val_net_stamp (Autodesk Fusion 360 design; units mm, degrees)
Autodesk Fusion 360 part; units mm, degrees
(part 1 of 3)
sketch "Sketch1" plane through (0, 0, 0) normal (0, 1, 0) x (1, 0, 0)
  spline S0 degree 3 poles (-44.0393, 3.3032) (-46.2975, 3.0854) (-48.3436, 1.4806) (-49.1116, -0.6573) knots 0 0 0 0 1 1 1 1
  spline S1 degree 3 poles (-49.1116, -0.6573) (-49.8911, -2.841) (-49.4211, -5.145) (-47.822, -6.9218) knots 0 0 0 0 1 1 1 1
  spline S2 degree 3 poles (-47.822, -6.9218) (-46.5783, -8.3031) (-45.6555, -10.4295) (-45.1168, -13.1405) knots 0 0 0 0 1 1 1 1
  line L0 (-45.1168, -13.1405) -> (-44.985, -13.7996)
  line L1 (-44.985, -13.7996) -> (-44.9563, -26.2082)
  line L2 (-44.9563, -26.2082) -> (-44.9276, -38.6169)
  line L3 (-44.9276, -38.6169) -> (-44.7729, -39.1958)
  spline S3 degree 3 poles (-44.7729, -39.1958) (-44.492, -40.2561) (-44.2227, -40.8636) (-43.6323, -41.7405) knots 0 0 0 0 1 1 1 1
  spline S4 degree 3 poles (-43.6323, -41.7405) (-42.6924, -43.1505) (-41.0761, -44.2968) (-39.4082, -44.7438) knots 0 0 0 0 1 1 1 1
  spline S5 degree 3 poles (-39.4082, -44.7438) (-38.474, -44.996) (-38.0384, -45.019) (-34.7829, -44.996) knots 0 0 0 0 1 1 1 1
  spline S6 degree 3 poles (-34.7829, -44.996) (-31.8599, -44.9731) (-31.728, -44.9674) (-31.3498, -44.847) knots 0 0 0 0 1 1 1 1
  spline S7 degree 3 poles (-31.3498, -44.847) (-30.8626, -44.6923) (-30.3124, -44.4401) (-29.957, -44.1994) knots 0 0 0 0 1 1 1 1
  spline S8 degree 3 poles (-29.957, -44.1994) (-29.8023, -44.1019) (-27.8077, -42.1475) (-25.5208, -39.8606) knots 0 0 0 0 1 1 1 1
  spline S9 degree 3 poles (-25.5208, -39.8606) (-23.2282, -37.5795) (-21.3311, -35.7168) (-21.3025, -35.7282) knots 0 0 0 0 1 1 1 1
  spline S10 degree 3 poles (-21.3025, -35.7282) (-21.2738, -35.7397) (-19.8868, -37.1267) (-18.2247, -38.806) knots 0 0 0 0 1 1 1 1
  line L4 (-18.2247, -38.806) -> (-15.1927, -41.8552)
  line L5 (-15.1927, -41.8552) -> (-18.1674, -41.8552)
  line L6 (-18.1674, -41.8552) -> (-21.142, -41.8552)
  line L7 (-21.142, -41.8552) -> (-22.7181, -43.4313)
  line L8 (-22.7181, -43.4313) -> (-24.2943, -45.0132)
  line L9 (-24.2943, -45.0132) -> (-14.2642, -44.9903)
  spline S11 degree 3 poles (-14.2642, -44.9903) (-4.3201, -44.9731) (-4.2284, -44.9731) (-3.7183, -44.8527) knots 0 0 0 0 1 1 1 1
  spline S12 degree 3 poles (-3.7183, -44.8527) (-0.9442, -44.2108) (1.0962, -42.3997) (1.9559, -39.832) knots 0 0 0 0 1 1 1 1
  spline S13 degree 3 poles (1.9559, -39.832) (2.3514, -38.6455) (2.3284, -39.4823) (2.3284, -26.4661) knots 0 0 0 0 1 1 1 1
  spline S14 degree 3 poles (2.3284, -26.4661) (2.3284, -18.5051) (2.3456, -14.5045) (2.3915, -14.0804) knots 0 0 0 0 1 1 1 1
  spline S15 degree 3 poles (2.3915, -14.0804) (2.5577, -12.3552) (3.1079, -10.4409) (3.8587, -8.9278) knots 0 0 0 0 1 1 1 1
  spline S16 degree 3 poles (3.8587, -8.9278) (4.2714, -8.1082) (4.6669, -7.5007) (5.2171, -6.8645) knots 0 0 0 0 1 1 1 1
  spline S17 degree 3 poles (5.2171, -6.8645) (5.9966, -5.9589) (6.3978, -5.2253) (6.6672, -4.228) knots 0 0 0 0 1 1 1 1
  spline S18 degree 3 poles (6.6672, -4.228) (6.799, -3.7236) (6.8162, -3.546) (6.8219, -2.7378) knots 0 0 0 0 1 1 1 1
  spline S19 degree 3 poles (6.8219, -2.7378) (6.8219, -1.9813) (6.8047, -1.7348) (6.7015, -1.3336) knots 0 0 0 0 1 1 1 1
  spline S20 degree 3 poles (6.7015, -1.3336) (5.7043, 2.6097) (1.2624, 4.5354) (-2.2109, 2.5351) knots 0 0 0 0 1 1 1 1
  spline S21 degree 3 poles (-2.2109, 2.5351) (-3.3572, 1.8703) (-4.7843, 1.3889) (-6.2975, 1.1596) knots 0 0 0 0 1 1 1 1
  spline S22 degree 3 poles (-6.2975, 1.1596) (-7.5756, 0.9647) (-8.9167, 0.9533) (-22.145, 0.9762) knots 0 0 0 0 1 1 1 1
  spline S23 degree 3 poles (-22.145, 0.9762) (-33.9862, 0.9934) (-35.2472, 1.0048) (-35.8948, 1.0908) knots 0 0 0 0 1 1 1 1
  spline S24 degree 3 poles (-35.8948, 1.0908) (-37.6888, 1.3373) (-39.2305, 1.8302) (-40.4915, 2.5695) knots 0 0 0 0 1 1 1 1
  spline S25 degree 3 poles (-40.4915, 2.5695) (-41.4945, 3.1541) (-42.807, 3.4235) (-44.0393, 3.3032) knots 0 0 0 0 1 1 1 1
  spline S26 degree 3 poles (-10.5731, -2.2678) (-7.352, -2.841) (-5.048, -4.3484) (-3.2196, -7.0937) knots 0 0 0 0 1 1 1 1
  spline S27 degree 3 poles (-3.2196, -7.0937) (-2.4975, -8.177) (-1.6607, -9.9939) (-1.3913, -11.0657) knots 0 0 0 0 1 1 1 1
  line L10 (-1.3913, -11.0657) -> (-1.3168, -11.3694)
  line L11 (-1.3168, -11.3694) -> (-4.3717, -14.4243)
  spline S28 degree 3 poles (-4.3717, -14.4243) (-7.0483, -17.1009) (-7.4151, -17.4906) (-7.3234, -17.5422) knots 0 0 0 0 1 1 1 1
  spline S29 degree 3 poles (-7.3234, -17.5422) (-7.1342, -17.6397) (-4.492, -18.7573) (-4.4519, -18.7573) knots 0 0 0 0 1 1 1 1
  spline S30 degree 3 poles (-4.4519, -18.7573) (-4.4233, -18.7573) (-3.6037, -17.9549) (-2.6293, -16.9805) knots 0 0 0 0 1 1 1 1
  spline S31 degree 3 poles (-2.6293, -16.9805) (-1.655, -16.0005) (-0.8354, -15.2038) (-0.8124, -15.2038) knots 0 0 0 0 1 1 1 1
  spline S32 degree 3 poles (-0.8124, -15.2038) (-0.7379, -15.2038) (-0.7551, -37.5336) (-0.8296, -38.0495) knots 0 0 0 0 1 1 1 1
  spline S33 degree 3 poles (-0.8296, -38.0495) (-1.0589, -39.7173) (-2.1708, -41.07) (-3.7871, -41.6488) knots 0 0 0 0 1 1 1 1
  line L12 (-3.7871, -41.6488) -> (-4.2914, -41.8265)
  line L13 (-4.2914, -41.8265) -> (-7.5584, -41.8437)
  line L14 (-7.5584, -41.8437) -> (-10.8196, -41.8609)
  line L15 (-10.8196, -41.8609) -> (-14.9921, -37.6884)
  line L16 (-14.9921, -37.6884) -> (-19.1646, -33.5159)
  line L17 (-19.1646, -33.5159) -> (-15.1411, -29.4924)
  spline S34 degree 3 poles (-15.1411, -29.4924) (-12.923, -27.2743) (-11.0947, -25.4689) (-11.0718, -25.4746) knots 0 0 0 0 1 1 1 1
  spline S35 degree 3 poles (-11.0718, -25.4746) (-11.0489, -25.4861) (-9.4842, -27.0336) (-7.5928, -28.9192) knots 0 0 0 0 1 1 1 1
  line L18 (-7.5928, -28.9192) -> (-4.1481, -32.3466)
  line L19 (-4.1481, -32.3466) -> (-4.1481, -30.1801)
  line L20 (-4.1481, -30.1801) -> (-4.1481, -28.0136)
  line L21 (-4.1481, -28.0136) -> (-11.6564, -20.5054)
  line L22 (-11.6564, -20.5054) -> (-19.1646, -12.9972)
  line L23 (-19.1646, -12.9972) -> (-15.4334, -9.266)
  line L24 (-15.4334, -9.266) -> (-11.7022, -5.5348)
  line L25 (-11.7022, -5.5348) -> (-12.6651, -5.5004)
  spline S36 degree 3 poles (-12.6651, -5.5004) (-13.1924, -5.4775) (-14.1496, -5.4603) (-14.7858, -5.4603) knots 0 0 0 0 1 1 1 1
  line L26 (-14.7858, -5.4603) -> (-15.955, -5.4603)
  line L27 (-15.955, -5.4603) -> (-18.6029, -8.1254)
  spline S37 degree 3 poles (-18.6029, -8.1254) (-20.053, -9.5927) (-21.2738, -10.7905) (-21.3082, -10.7905) knots 0 0 0 0 1 1 1 1
  spline S38 degree 3 poles (-21.3082, -10.7905) (-21.3426, -10.7905) (-22.3743, -9.7933) (-23.6008, -8.5667) knots 0 0 0 0 1 1 1 1
  spline S39 degree 3 poles (-23.6008, -8.5667) (-24.8216, -7.3459) (-25.8361, -6.3716) (-25.8475, -6.406) knots 0 0 0 0 1 1 1 1
  spline S40 degree 3 poles (-25.8475, -6.406) (-25.8647, -6.4346) (-26.157, -7.1224) (-26.5009, -7.9248) knots 0 0 0 0 1 1 1 1
  line L28 (-26.5009, -7.9248) -> (-27.1257, -9.3863)
  line L29 (-27.1257, -9.3863) -> (-20.1791, -16.3329)
  line L30 (-20.1791, -16.3329) -> (-13.2325, -23.2852)
  line L31 (-13.2325, -23.2852) -> (-17.2732, -27.3259)
  line L32 (-17.2732, -27.3259) -> (-21.3139, -31.3666)
  line L33 (-21.3139, -31.3666) -> (-23.5607, -29.1198)
  line L34 (-23.5607, -29.1198) -> (-25.8074, -26.8731)
  line L35 (-25.8074, -26.8731) -> (-25.9278, -27.1597)
  spline S41 degree 3 poles (-25.9278, -27.1597) (-25.9966, -27.3144) (-26.2831, -27.9907) (-26.5697, -28.6613) knots 0 0 0 0 1 1 1 1
  line L36 (-26.5697, -28.6613) -> (-27.0913, -29.8878)
  line L37 (-27.0913, -29.8878) -> (-25.3088, -31.6703)
  spline S42 degree 3 poles (-25.3088, -31.6703) (-24.323, -32.6561) (-23.5206, -33.4872) (-23.5206, -33.5159) knots 0 0 0 0 1 1 1 1
  spline S43 degree 3 poles (-23.5206, -33.5159) (-23.5206, -33.5503) (-25.3088, -35.3557) (-27.4867, -37.5336) knots 0 0 0 0 1 1 1 1
  spline S44 degree 3 poles (-27.4867, -37.5336) (-31.195, -41.2304) (-31.4816, -41.4998) (-31.8312, -41.6603) knots 0 0 0 0 1 1 1 1
  line L38 (-31.8312, -41.6603) -> (-32.2037, -41.8265)
  line L39 (-32.2037, -41.8265) -> (-35.0924, -41.8437)
  spline S45 degree 3 poles (-35.0924, -41.8437) (-38.3708, -41.8609) (-38.4568, -41.8494) (-39.3681, -41.4024) knots 0 0 0 0 1 1 1 1
  spline S46 degree 3 poles (-39.3681, -41.4024) (-40.4399, -40.8694) (-41.185, -40.0039) (-41.6148, -38.7888) knots 0 0 0 0 1 1 1 1
  line L40 (-41.6148, -38.7888) -> (-41.7753, -38.3303)
  line L41 (-41.7753, -38.3303) -> (-41.7925, -26.7928)
  spline S47 degree 3 poles (-41.7925, -26.7928) (-41.7982, -20.4538) (-41.7868, -15.2611) (-41.7639, -15.2611) knots 0 0 0 0 1 1 1 1
  spline S48 degree 3 poles (-41.7639, -15.2611) (-41.6951, -15.2611) (-33.7799, -23.1877) (-33.7799, -23.2565) knots 0 0 0 0 1 1 1 1
  spline S49 degree 3 poles (-33.7799, -23.2565) (-33.7799, -23.2909) (-34.8345, -24.3742) (-36.1298, -25.6637) knots 0 0 0 0 1 1 1 1
  line L42 (-36.1298, -25.6637) -> (-38.4797, -28.0136)
  line L43 (-38.4797, -28.0136) -> (-38.4797, -30.1801)
  line L44 (-38.4797, -30.1801) -> (-38.4797, -32.3466)
  line L45 (-38.4797, -32.3466) -> (-32.0261, -25.8701)
  spline S50 degree 3 poles (-32.0261, -25.8701) (-28.4783, -22.3108) (-25.5724, -19.3763) (-25.5724, -19.3534) knots 0 0 0 0 1 1 1 1
  spline S51 degree 3 poles (-25.5724, -19.3534) (-25.5724, -19.3133) (-27.5956, -18.4249) (-28.3235, -18.144) knots 0 0 0 0 1 1 1 1
  line L46 (-28.3235, -18.144) -> (-28.5757, -18.0523)
  line L47 (-28.5757, -18.0523) -> (-30.0888, -19.5654)
  line L48 (-30.0888, -19.5654) -> (-31.6019, -21.0786)
  line L49 (-31.6019, -21.0786) -> (-36.4508, -16.2297)
  line L50 (-36.4508, -16.2297) -> (-41.2939, -11.3866)
  line L51 (-41.2939, -11.3866) -> (-41.1105, -10.8192)
  spline S52 degree 3 poles (-41.1105, -10.8192) (-40.5087, -8.9278) (-39.6203, -7.2542) (-38.5141, -5.9303) knots 0 0 0 0 1 1 1 1
  spline S53 degree 3 poles (-38.5141, -5.9303) (-37.9868, -5.2941) (-37.1615, -4.526) (-36.5024, -4.0503) knots 0 0 0 0 1 1 1 1
  spline S54 degree 3 poles (-36.5024, -4.0503) (-35.8891, -3.6147) (-34.588, -2.9499) (-33.8659, -2.7149) knots 0 0 0 0 1 1 1 1
  spline S55 degree 3 poles (-33.8659, -2.7149) (-33.1896, -2.4914) (-32.0031, -2.2506) (-31.2867, -2.1933) knots 0 0 0 0 1 1 1 1
  spline S56 degree 3 poles (-31.2867, -2.1933) (-30.9715, -2.1704) (-26.3003, -2.1532) (-20.9127, -2.1647) knots 0 0 0 0 1 1 1 1
  spline S57 degree 3 poles (-20.9127, -2.1647) (-12.0748, -2.1704) (-11.0603, -2.1819) (-10.5731, -2.2678) knots 0 0 0 0 1 1 1 1
extrude "Extrude1" add sketch "Sketch1" against normal blind 12 makes body 1
sketch "Sketch2" plane through (0, 0, 0) normal (0, 1, 0) x (1, 0, 0)
  spline S0 degree 3 poles (34.0518, 3.2009) (31.7591, 2.9797) (29.6817, 1.3504) (28.902, -0.8201) knots 0 0 0 0 1 1 1 1
  spline S1 degree 3 poles (28.902, -0.8201) (28.1106, -3.0372) (28.5877, -5.3764) (30.2112, -7.1803) knots 0 0 0 0 1 1 1 1
  spline S2 degree 3 poles (30.2112, -7.1803) (31.474, -8.5827) (32.4108, -10.7416) (32.9578, -13.494) knots 0 0 0 0 1 1 1 1
  line L0 (32.9578, -13.494) -> (33.0917, -14.1632)
  line L1 (33.0917, -14.1632) -> (33.1208, -26.7614)
  line L2 (33.1208, -26.7614) -> (33.1499, -39.3597)
  line L3 (33.1499, -39.3597) -> (33.307, -39.9474)
  spline S3 degree 3 poles (33.307, -39.9474) (33.5921, -41.0239) (33.8656, -41.6407) (34.465, -42.531) knots 0 0 0 0 1 1 1 1
  spline S4 degree 3 poles (34.465, -42.531) (35.4193, -43.9625) (37.0603, -45.1263) (38.7536, -45.5802) knots 0 0 0 0 1 1 1 1
  spline S5 degree 3 poles (38.7536, -45.5802) (39.7021, -45.8363) (40.1444, -45.8595) (43.4496, -45.8363) knots 0 0 0 0 1 1 1 1
  spline S6 degree 3 poles (43.4496, -45.8363) (46.4173, -45.813) (46.5511, -45.8072) (46.9352, -45.685) knots 0 0 0 0 1 1 1 1
  spline S7 degree 3 poles (46.9352, -45.685) (47.4298, -45.5278) (47.9884, -45.2718) (48.3492, -45.0274) knots 0 0 0 0 1 1 1 1
  spline S8 degree 3 poles (48.3492, -45.0274) (48.5063, -44.9285) (50.5313, -42.9442) (52.8531, -40.6224) knots 0 0 0 0 1 1 1 1
  spline S9 degree 3 poles (52.8531, -40.6224) (55.1808, -38.3064) (57.1069, -36.4152) (57.136, -36.4269) knots 0 0 0 0 1 1 1 1
  spline S10 degree 3 poles (57.136, -36.4269) (57.1651, -36.4385) (58.5733, -37.8467) (60.2608, -39.5517) knots 0 0 0 0 1 1 1 1
  line L4 (60.2608, -39.5517) -> (63.3391, -42.6474)
  line L5 (63.3391, -42.6474) -> (60.319, -42.6474)
  line L6 (60.319, -42.6474) -> (57.2989, -42.6474)
  line L7 (57.2989, -42.6474) -> (55.6987, -44.2477)
  line L8 (55.6987, -44.2477) -> (54.0984, -45.8537)
  line L9 (54.0984, -45.8537) -> (64.2818, -45.8304)
  spline S11 degree 3 poles (64.2818, -45.8304) (74.3778, -45.813) (74.4709, -45.813) (74.9888, -45.6908) knots 0 0 0 0 1 1 1 1
  spline S12 degree 3 poles (74.9888, -45.6908) (77.8052, -45.039) (79.8768, -43.2002) (80.7497, -40.5933) knots 0 0 0 0 1 1 1 1
  spline S13 degree 3 poles (80.7497, -40.5933) (81.1512, -39.3887) (81.1279, -40.2383) (81.1279, -27.0233) knots 0 0 0 0 1 1 1 1
  spline S14 degree 3 poles (81.1279, -27.0233) (81.1279, -18.9406) (81.1454, -14.8789) (81.1919, -14.4483) knots 0 0 0 0 1 1 1 1
  spline S15 degree 3 poles (81.1919, -14.4483) (81.3607, -12.6968) (81.9193, -10.7532) (82.6816, -9.217) knots 0 0 0 0 1 1 1 1
  spline S16 degree 3 poles (82.6816, -9.217) (83.1006, -8.3849) (83.5021, -7.768) (84.0607, -7.1221) knots 0 0 0 0 1 1 1 1
  spline S17 degree 3 poles (84.0607, -7.1221) (84.8521, -6.2027) (85.2594, -5.4579) (85.5329, -4.4454) knots 0 0 0 0 1 1 1 1
  spline S18 degree 3 poles (85.5329, -4.4454) (85.6668, -3.9333) (85.6842, -3.7529) (85.69, -2.9324) knots 0 0 0 0 1 1 1 1
  spline S19 degree 3 poles (85.69, -2.9324) (85.69, -2.1643) (85.6726, -1.9141) (85.5678, -1.5068) knots 0 0 0 0 1 1 1 1
  spline S20 degree 3 poles (85.5678, -1.5068) (84.5553, 2.4967) (80.0456, 4.4519) (76.5192, 2.4211) knots 0 0 0 0 1 1 1 1
  spline S21 degree 3 poles (76.5192, 2.4211) (75.3554, 1.7461) (73.9065, 1.2573) (72.3702, 1.0245) knots 0 0 0 0 1 1 1 1
  spline S22 degree 3 poles (72.3702, 1.0245) (71.0726, 0.8267) (69.7109, 0.815) (56.2806, 0.8383) knots 0 0 0 0 1 1 1 1
  spline S23 degree 3 poles (56.2806, 0.8383) (44.2584, 0.8558) (42.9782, 0.8674) (42.3207, 0.9547) knots 0 0 0 0 1 1 1 1
  spline S24 degree 3 poles (42.3207, 0.9547) (40.4993, 1.2049) (38.934, 1.7054) (37.6538, 2.456) knots 0 0 0 0 1 1 1 1
  spline S25 degree 3 poles (37.6538, 2.456) (36.6355, 3.0496) (35.3029, 3.3231) (34.0518, 3.2009) knots 0 0 0 0 1 1 1 1
  spline S26 degree 3 poles (68.0292, -2.4553) (71.2995, -3.0372) (73.6388, -4.5676) (75.4951, -7.3549) knots 0 0 0 0 1 1 1 1
  spline S27 degree 3 poles (75.4951, -7.3549) (76.2283, -8.4547) (77.0778, -10.2993) (77.3513, -11.3875) knots 0 0 0 0 1 1 1 1
  line L10 (77.3513, -11.3875) -> (77.427, -11.6959)
  line L11 (77.427, -11.6959) -> (74.3254, -14.7975)
  spline S28 degree 3 poles (74.3254, -14.7975) (71.6079, -17.515) (71.2355, -17.9106) (71.3286, -17.963) knots 0 0 0 0 1 1 1 1
  spline S29 degree 3 poles (71.3286, -17.963) (71.5206, -18.0619) (74.2032, -19.1967) (74.244, -19.1967) knots 0 0 0 0 1 1 1 1
  spline S30 degree 3 poles (74.244, -19.1967) (74.2731, -19.1967) (75.1052, -18.382) (76.0944, -17.3928) knots 0 0 0 0 1 1 1 1
  spline S31 degree 3 poles (76.0944, -17.3928) (77.0837, -16.3977) (77.9158, -15.5888) (77.9391, -15.5888) knots 0 0 0 0 1 1 1 1
  spline S32 degree 3 poles (77.9391, -15.5888) (78.0147, -15.5888) (77.9972, -38.2599) (77.9216, -38.7836) knots 0 0 0 0 1 1 1 1
  spline S33 degree 3 poles (77.9216, -38.7836) (77.6888, -40.4769) (76.5599, -41.8502) (74.919, -42.4379) knots 0 0 0 0 1 1 1 1
  line L12 (74.919, -42.4379) -> (74.4069, -42.6183)
  line L13 (74.4069, -42.6183) -> (71.09, -42.6358)
  line L14 (71.09, -42.6358) -> (67.779, -42.6532)
  line L15 (67.779, -42.6532) -> (63.5427, -38.417)
  line L16 (63.5427, -38.417) -> (59.3065, -34.1807)
  line L17 (59.3065, -34.1807) -> (63.3914, -30.0957)
  spline S34 degree 3 poles (63.3914, -30.0957) (65.6434, -27.8438) (67.4997, -26.0108) (67.523, -26.0166) knots 0 0 0 0 1 1 1 1
  spline S35 degree 3 poles (67.523, -26.0166) (67.5462, -26.0282) (69.1348, -27.5994) (71.0551, -29.5138) knots 0 0 0 0 1 1 1 1
  line L18 (71.0551, -29.5138) -> (74.5524, -32.9936)
  line L19 (74.5524, -32.9936) -> (74.5524, -30.794)
  line L20 (74.5524, -30.794) -> (74.5524, -28.5944)
  line L21 (74.5524, -28.5944) -> (66.9294, -20.9715)
  line L22 (66.9294, -20.9715) -> (59.3065, -13.3485)
  line L23 (59.3065, -13.3485) -> (63.0947, -9.5603)
  line L24 (63.0947, -9.5603) -> (66.8829, -5.7721)
  line L25 (66.8829, -5.7721) -> (65.9053, -5.7372)
  spline S36 degree 3 poles (65.9053, -5.7372) (65.3699, -5.7139) (64.3981, -5.6965) (63.7522, -5.6965) knots 0 0 0 0 1 1 1 1
  line L26 (63.7522, -5.6965) -> (62.5651, -5.6965)
  line L27 (62.5651, -5.6965) -> (59.8767, -8.4023)
  spline S37 degree 3 poles (59.8767, -8.4023) (58.4045, -9.892) (57.1651, -11.1082) (57.1301, -11.1082) knots 0 0 0 0 1 1 1 1
  spline S38 degree 3 poles (57.1301, -11.1082) (57.0952, -11.1082) (56.0478, -10.0957) (54.8025, -8.8504) knots 0 0 0 0 1 1 1 1
  spline S39 degree 3 poles (54.8025, -8.8504) (53.5631, -7.6109) (52.5331, -6.6217) (52.5215, -6.6566) knots 0 0 0 0 1 1 1 1
  spline S40 degree 3 poles (52.5215, -6.6566) (52.504, -6.6857) (52.2072, -7.384) (51.8581, -8.1987) knots 0 0 0 0 1 1 1 1
  line L28 (51.8581, -8.1987) -> (51.2238, -9.6825)
  line L29 (51.2238, -9.6825) -> (58.2765, -16.7352)
  line L30 (58.2765, -16.7352) -> (65.3292, -23.7937)
  line L31 (65.3292, -23.7937) -> (61.2268, -27.8961)
  line L32 (61.2268, -27.8961) -> (57.1243, -31.9986)
  line L33 (57.1243, -31.9986) -> (54.8433, -29.7175)
  line L34 (54.8433, -29.7175) -> (52.5622, -27.4364)
  line L35 (52.5622, -27.4364) -> (52.44, -27.7274)
  spline S41 degree 3 poles (52.44, -27.7274) (52.3702, -27.8845) (52.0792, -28.5711) (51.7883, -29.252) knots 0 0 0 0 1 1 1 1
  line L36 (51.7883, -29.252) -> (51.2587, -30.4972)
  line L37 (51.2587, -30.4972) -> (53.0685, -32.307)
  spline S42 degree 3 poles (53.0685, -32.307) (54.0693, -33.3078) (54.884, -34.1516) (54.884, -34.1807) knots 0 0 0 0 1 1 1 1
  spline S43 degree 3 poles (54.884, -34.1807) (54.884, -34.2156) (53.0685, -36.0486) (50.8572, -38.2599) knots 0 0 0 0 1 1 1 1
  spline S44 degree 3 poles (50.8572, -38.2599) (47.0923, -42.0131) (46.8013, -42.2866) (46.4464, -42.4496) knots 0 0 0 0 1 1 1 1
  line L38 (46.4464, -42.4496) -> (46.0681, -42.6183)
  line L39 (46.0681, -42.6183) -> (43.1353, -42.6358)
  spline S45 degree 3 poles (43.1353, -42.6358) (39.8068, -42.6532) (39.7196, -42.6416) (38.7943, -42.1877) knots 0 0 0 0 1 1 1 1
  spline S46 degree 3 poles (38.7943, -42.1877) (37.7062, -41.6465) (36.9497, -40.7679) (36.5133, -39.5342) knots 0 0 0 0 1 1 1 1
  line L40 (36.5133, -39.5342) -> (36.3503, -39.0687)
  line L41 (36.3503, -39.0687) -> (36.3329, -27.355)
  spline S47 degree 3 poles (36.3329, -27.355) (36.3271, -20.9191) (36.3387, -15.647) (36.362, -15.647) knots 0 0 0 0 1 1 1 1
  spline S48 degree 3 poles (36.362, -15.647) (36.4318, -15.647) (44.4679, -23.6948) (44.4679, -23.7646) knots 0 0 0 0 1 1 1 1
  spline S49 degree 3 poles (44.4679, -23.7646) (44.4679, -23.7995) (43.3972, -24.8993) (42.0821, -26.2086) knots 0 0 0 0 1 1 1 1
  line L42 (42.0821, -26.2086) -> (39.6963, -28.5944)
  line L43 (39.6963, -28.5944) -> (39.6963, -30.794)
  line L44 (39.6963, -30.794) -> (39.6963, -32.9936)
  line L45 (39.6963, -32.9936) -> (46.2485, -26.4181)
  spline S50 degree 3 poles (46.2485, -26.4181) (49.8505, -22.8045) (52.8008, -19.8251) (52.8008, -19.8018) knots 0 0 0 0 1 1 1 1
  spline S51 degree 3 poles (52.8008, -19.8018) (52.8008, -19.7611) (50.7467, -18.8592) (50.0076, -18.574) knots 0 0 0 0 1 1 1 1
  line L46 (50.0076, -18.574) -> (49.7516, -18.4809)
  line L47 (49.7516, -18.4809) -> (48.2154, -20.0171)
  line L48 (48.2154, -20.0171) -> (46.6791, -21.5534)
  line L49 (46.6791, -21.5534) -> (41.7562, -16.6305)
  line L50 (41.7562, -16.6305) -> (36.8391, -11.7134)
  line L51 (36.8391, -11.7134) -> (37.0253, -11.1373)
  spline S52 degree 3 poles (37.0253, -11.1373) (37.6363, -9.217) (38.5383, -7.5178) (39.6614, -6.1736) knots 0 0 0 0 1 1 1 1
  spline S53 degree 3 poles (39.6614, -6.1736) (40.1967, -5.5277) (41.0347, -4.748) (41.7039, -4.265) knots 0 0 0 0 1 1 1 1
  spline S54 degree 3 poles (41.7039, -4.265) (42.3265, -3.8227) (43.6474, -3.1477) (44.3806, -2.9091) knots 0 0 0 0 1 1 1 1
  spline S55 degree 3 poles (44.3806, -2.9091) (45.0673, -2.6822) (46.2718, -2.4378) (46.9992, -2.3796) knots 0 0 0 0 1 1 1 1
  spline S56 degree 3 poles (46.9992, -2.3796) (47.3192, -2.3563) (52.0618, -2.3389) (57.5317, -2.3505) knots 0 0 0 0 1 1 1 1
  spline S57 degree 3 poles (57.5317, -2.3505) (66.5046, -2.3563) (67.5346, -2.368) (68.0292, -2.4553) knots 0 0 0 0 1 1 1 1
  line L52 (28.5927, -14.6139) -> (28.6208, -26.7718)
  line L53 (28.6208, -26.7718) -> (28.6512, -39.9559)
  line L54 (28.6512, -39.9559) -> (28.9596, -41.1095)
  spline S58 degree 3 poles (28.9596, -41.1095) (29.1624, -41.8737) (29.4207, -42.6577) (29.7867, -43.4188) (30.0662, -43.9999) (30.3895, -44.5347) (30.7268, -45.0362) knots 0.002463 0.002463 0.002463 0.002463 0.566846 0.566846 0.566846 0.997755 0.997755 0.997755 0.997755
  spline S59 degree 3 poles (30.7268, -45.0362) (31.8623, -46.7358) (33.3627, -48.0126) (35.086, -48.9323) (35.8654, -49.3483) (36.6957, -49.6868) (37.5808, -49.9247) knots 0.001217 0.001217 0.001217 0.001217 0.688337 0.688337 0.688337 0.9991 0.9991 0.9991 0.9991
  spline S60 degree 3 poles (37.5809, -49.9247) (38.1393, -50.0755) (38.9538, -50.2376) (39.748, -50.2925) (40.6559, -50.3552) (41.5987, -50.3487) (43.2784, -50.3375) knots 0 0 0 0 0.456967 0.456967 0.456967 0.979343 0.979343 0.979343 0.979343
  line L55 (43.2784, -50.3375) -> (43.2375, -50.3785)
  line L56 (43.2375, -50.3785) -> (64.2895, -50.3304)
  spline S61 degree 3 poles (64.2895, -50.3304) (69.3375, -50.3217) (71.8718, -50.3178) (73.2853, -50.2995) (73.992, -50.2904) (74.4136, -50.2812) (74.8445, -50.2498) (75.1344, -50.2286) (75.4759, -50.185) (75.7431, -50.1318) (75.8658, -50.1074) (75.9593, -50.0853) (76.0131, -50.0726) knots 0 0 0 0 0.5 0.5 0.5 0.75 0.75 0.75 0.918213 0.918213 0.918213 0.99543 0.99543 0.99543 0.99543
  spline S62 degree 3 poles (76.0131, -50.0726) (78.7497, -49.4373) (81.2312, -47.9496) (82.9657, -45.7927) (83.8624, -44.6776) (84.5567, -43.3962) (85.0168, -42.022) (85.0171, -42.0211) (85.0175, -42.0201) (85.0178, -42.0192) knots 0.000788 0.000788 0.000788 0.000788 0.659473 0.659473 0.659473 1 1 1 1.000365 1.000365 1.000365 1.000365
  spline S63 degree 3 poles (85.0178, -42.0192) (85.0181, -42.0182) (85.0184, -42.0173) (85.0187, -42.0163) (85.0516, -41.9176) (85.1158, -41.7567) (85.2177, -41.4143) (85.3321, -41.0296) (85.439, -40.5049) (85.4918, -40.0367) (85.5914, -39.1525) (85.6029, -38.2865) (85.6162, -36.5721) (85.6311, -34.6649) (85.6279, -31.7431) (85.6279, -27.0233) knots -0.000791 -0.000791 -0.000791 -0.000791 0 0 0 0.151411 0.151411 0.151411 0.321524 0.321524 0.321524 0.642699 0.642699 0.642699 1 1 1 1
  spline S64 degree 3 poles (85.6279, -27.0233) (85.6279, -23.1991) (85.6318, -20.2771) (85.6408, -18.2245) (85.6454, -17.1759) (85.6514, -16.3534) (85.6586, -15.7622) (85.664, -15.321) (85.6707, -15.0001) (85.6757, -14.8547) (85.6761, -14.8429) (85.6765, -14.8324) (85.6768, -14.8233) knots 0 0 0 0 0.473518 0.473518 0.473518 0.715422 0.715422 0.715422 0.895914 0.895914 0.895914 0.91057 0.91057 0.91057 0.91057
  spline S65 degree 3 poles (85.6768, -14.8233) (85.78, -13.825) (86.1372, -12.4963) (86.5583, -11.5465) (86.6077, -11.435) (86.6576, -11.3286) (86.707, -11.2286) knots 0.016663 0.016663 0.016663 0.016663 0.893157 0.893157 0.893157 0.99609 0.99609 0.99609 0.99609
  spline S66 degree 3 poles (86.707, -11.2286) (87.0043, -10.6397) (87.1373, -10.444) (87.4643, -10.0658) (87.4655, -10.0645) (87.4666, -10.0631) (87.4678, -10.0618) knots 0.006764 0.006764 0.006764 0.006764 1 1 1 1.002067 1.002067 1.002067 1.002067
  spline S67 degree 3 poles (87.4678, -10.0618) (87.4689, -10.0605) (87.4701, -10.0591) (87.4712, -10.0578) (88.1686, -9.2476) (88.815, -8.3206) (89.28, -7.2967) (89.5333, -6.7388) (89.7284, -6.1697) (89.8772, -5.6188) (89.8788, -5.6129) (89.8804, -5.607) (89.882, -5.6011) knots -0.001455 -0.001455 -0.001455 -0.001455 0 0 0 0.647342 0.647342 0.647342 1 1 1 1.005845 1.005845 1.005845 1.005845
  spline S68 degree 3 poles (89.882, -5.6011) (89.8836, -5.5951) (89.8851, -5.5892) (89.8867, -5.5833) (89.9571, -5.3137) (90.0431, -4.9596) (90.1002, -4.5568) (90.1621, -4.1205) (90.1782, -3.7263) (90.185, -3.3701) (90.1876, -3.2384) (90.1889, -3.1062) (90.1899, -2.9643) (90.19, -2.959) (90.19, -2.9537) (90.19, -2.9484) knots -0.011583 -0.011583 -0.011583 -0.011583 0 0 0 0.402629 0.402629 0.402629 0.838702 0.838702 0.838702 1 1 1 1.006483 1.006483 1.006483 1.006483
  spline S69 degree 3 poles (90.19, -2.9484) (90.19, -2.9431) (90.19, -2.9377) (90.19, -2.9324) (90.19, -2.4687) (90.1909, -2.0734) (90.1389, -1.562) (90.0975, -1.1547) (90.0104, -0.7153) (89.9283, -0.3949) knots -0.006925 -0.006925 -0.006925 -0.006925 0 0 0 0.554445 0.554445 0.554445 0.995951 0.995951 0.995951 0.995951
  spline S70 degree 3 poles (89.9283, -0.3949) (89.2588, 2.2434) (87.6414, 4.4379) (85.5824, 5.8498) (83.3601, 7.3736) (80.5963, 8.0488) (77.8293, 7.5933) (76.6106, 7.3927) (75.3981, 6.9683) (74.2734, 6.3206) (74.2714, 6.3195) (74.2694, 6.3184) (74.2674, 6.3172) knots 0.000423 0.000423 0.000423 0.000423 0.3917 0.3917 0.3917 0.814004 0.814004 0.814004 1 1 1 1.000565 1.000565 1.000565 1.000565
  spline S71 degree 3 poles (74.2674, 6.3172) (74.2655, 6.316) (74.2635, 6.3149) (74.2615, 6.3137) (73.6843, 5.979) (72.7241, 5.6295) (71.6961, 5.4737) (71.6954, 5.4736) (71.6947, 5.4735) (71.694, 5.4734) knots -0.00171 -0.00171 -0.00171 -0.00171 0 0 0 1 1 1 1.000449 1.000449 1.000449 1.000449
  spline S72 degree 3 poles (71.694, 5.4734) (71.6933, 5.4733) (71.6927, 5.4732) (71.692, 5.4731) (71.4636, 5.4383) (71.3375, 5.4212) (70.8719, 5.3978) (69.9429, 5.351) (67.867, 5.3283) (63.1123, 5.3297) (61.2764, 5.3303) (59.0354, 5.3336) (56.2884, 5.3383) (56.2882, 5.3383) (56.2879, 5.3383) (56.2877, 5.3383) knots -0.000531 -0.000531 -0.000531 -0.000531 0 0 0 0.265563 0.265563 0.265563 0.795413 0.795413 0.795413 1 1 1 1.000016 1.000016 1.000016 1.000016
  spline S73 degree 3 poles (56.2877, 5.3383) (56.2875, 5.3383) (56.2873, 5.3383) (56.2871, 5.3383) (49.133, 5.3487) (45.769, 5.3576) (44.1594, 5.38) (43.3075, 5.3919) (42.958, 5.4118) (42.9119, 5.4159) (42.911, 5.416) (42.9103, 5.416) (42.9096, 5.4161) knots -0.000018 -0.000018 -0.000018 -0.000018 0 0 0 0.595196 0.595196 0.595196 0.910216 0.910216 0.910216 0.916088 0.916088 0.916088 0.916088
  spline S74 degree 3 poles (42.9096, 5.4161) (41.5575, 5.6043) (40.5785, 5.9576) (39.93, 6.3379) (39.9283, 6.3389) (39.9266, 6.3399) (39.9249, 6.3409) knots 0.005759 0.005759 0.005759 0.005759 1 1 1 1.001321 1.001321 1.001321 1.001321
  spline S75 degree 3 poles (39.9249, 6.3409) (39.9232, 6.3419) (39.9215, 6.3428) (39.9198, 6.3438) (38.3615, 7.2521) (36.7048, 7.6682) (34.9959, 7.7237) (34.5397, 7.7385) (34.079, 7.7249) (33.6144, 7.6795) knots -0.001663 -0.001663 -0.001663 -0.001663 0 0 0 0.789303 0.789303 0.789303 1 1 1 1
  spline S76 degree 3 poles (33.6144, 7.6795) (31.0087, 7.4269) (28.7159, 6.2217) (27.0024, 4.4425) (25.9971, 3.3987) (25.1834, 2.1388) (24.6669, 0.7013) (24.6659, 0.6984) (24.6649, 0.6956) (24.6639, 0.6927) knots 0.000439 0.000439 0.000439 0.000439 0.630416 0.630416 0.630416 1 1 1 1.001322 1.001322 1.001322 1.001322
  spline S77 degree 3 poles (24.6639, 0.6927) (23.792, -1.7499) (23.8315, -4.463) (24.7752, -6.841) (25.2611, -8.0655) (25.9744, -9.1996) (26.8664, -10.1907) (26.8665, -10.1908) (26.8666, -10.1909) (26.8668, -10.1911) knots 0 0 0 0 0.660104 0.660104 0.660104 1 1 1 1.000071 1.000071 1.000071 1.000071
  spline S78 degree 3 poles (26.8668, -10.1911) (26.8669, -10.1912) (26.867, -10.1913) (26.8671, -10.1914) (27.2467, -10.6131) (27.8393, -11.6247) (28.2707, -13.2034) (28.3696, -13.5653) (28.4615, -13.9552) (28.5441, -14.3711) (28.5443, -14.372) (28.5445, -14.3729) (28.5447, -14.3738) knots -0.000091 -0.000091 -0.000091 -0.000091 0 0 0 0.813499 0.813499 0.813499 1 1 1 1.000326 1.000326 1.000326 1.000326
  line L57 (28.5447, -14.3738) -> (28.5927, -14.6139)
  spline S79 degree 3 poles (28.1853, -41.3106) (28.3952, -42.1024) (28.6708, -42.9432) (29.0632, -43.7602) (29.3636, -44.3856) (29.7101, -44.9579) (30.0622, -45.4817) knots 0.001492 0.001492 0.001492 0.001492 0.565614 0.565614 0.565614 0.997484 0.997484 0.997484 0.997484
  spline S80 degree 3 poles (30.0622, -45.4817) (31.2338, -47.2348) (32.7505, -48.5474) (34.4897, -49.5182) (35.3819, -50.0162) (36.3395, -50.4194) (37.3724, -50.6971) knots 0.001343 0.001343 0.001343 0.001343 0.660747 0.660747 0.660747 0.999011 0.999011 0.999011 0.999011
  spline S81 degree 3 poles (37.3724, -50.6971) (37.9297, -50.8475) (38.7865, -51.022) (39.592, -51.0832) (40.1427, -51.1251) (40.6793, -51.137) (41.348, -51.1415) knots 0 0 0 0 0.438651 0.438651 0.438651 0.73853 0.73853 0.73853 0.73853
  line L58 (41.348, -51.1415) -> (41.3067, -51.183)
  line L59 (41.3067, -51.183) -> (64.2909, -51.1304)
  spline S82 degree 3 poles (64.2909, -51.1304) (69.3389, -51.1217) (71.8708, -51.1179) (73.2956, -51.0994) (74.008, -51.0902) (74.4377, -51.0816) (74.9027, -51.0476) (75.1922, -51.0265) (75.5363, -50.9854) (75.8301, -50.9298) (75.9985, -50.898) (76.1292, -50.8672) (76.1953, -50.8516) knots 0 0 0 0 0.5 0.5 0.5 0.75 0.75 0.75 0.905652 0.905652 0.905652 0.994872 0.994872 0.994872 0.994872
  spline S83 degree 3 poles (76.1953, -50.8516) (78.9721, -50.2067) (81.5254, -48.7257) (83.3624, -46.568) (84.4288, -45.3154) (85.2484, -43.8501) (85.7754, -42.276) (85.7758, -42.2749) (85.7762, -42.2738) (85.7766, -42.2727) knots 0.000881 0.000881 0.000881 0.000881 0.63304 0.63304 0.63304 1 1 1 1.00043 1.00043 1.00043 1.00043
  spline S84 degree 3 poles (85.7766, -42.2727) (85.7769, -42.2715) (85.7773, -42.2704) (85.7777, -42.2693) (85.8042, -42.1896) (85.8632, -42.0409) (85.9679, -41.6972) (86.0879, -41.3033) (86.2125, -40.7327) (86.2734, -40.2394) (86.3894, -39.3) (86.3986, -38.4761) (86.4136, -36.8869) (86.4315, -34.9791) (86.4279, -32.0037) (86.4279, -27.0233) knots -0.000931 -0.000931 -0.000931 -0.000931 0 0 0 0.143922 0.143922 0.143922 0.308857 0.308857 0.308857 0.622947 0.622947 0.622947 1 1 1 1
  spline S85 degree 3 poles (86.4279, -27.0233) (86.4279, -23.225) (86.4318, -20.3172) (86.4406, -18.269) (86.4452, -17.2152) (86.4511, -16.388) (86.4583, -15.7942) (86.4636, -15.3508) (86.4703, -15.028) (86.475, -14.8883) (86.4751, -14.8853) (86.4752, -14.8824) (86.4753, -14.8796) knots 0 0 0 0 0.470371 0.470371 0.470371 0.712378 0.712378 0.712378 0.893105 0.893105 0.893105 0.896967 0.896967 0.896967 0.896967
  spline S86 degree 3 poles (86.4753, -14.8796) (86.5675, -14.0165) (86.8785, -12.8313) (87.2426, -11.9789) (87.3027, -11.838) (87.3635, -11.706) (87.4227, -11.5861) knots 0.025015 0.025015 0.025015 0.025015 0.857358 0.857358 0.857358 0.994911 0.994911 0.994911 0.994911
  spline S87 degree 3 poles (87.4227, -11.5861) (87.6698, -11.0971) (87.7701, -10.9505) (87.9887, -10.6847) (88.0135, -10.6546) (88.0403, -10.6228) (88.0694, -10.5891) (88.0708, -10.5876) (88.0721, -10.586) (88.0735, -10.5844) knots 0.008653 0.008653 0.008653 0.008653 0.898949 0.898949 0.898949 1 1 1 1.002435 1.002435 1.002435 1.002435
  spline S88 degree 3 poles (88.0735, -10.5844) (88.0749, -10.5828) (88.0762, -10.5813) (88.0776, -10.5797) (88.7711, -9.7739) (89.436, -8.8374) (89.9313, -7.7935) (90.2416, -7.1395) (90.4769, -6.4667) (90.6495, -5.8275) (90.6514, -5.8205) (90.6533, -5.8135) (90.6552, -5.8065) knots -0.001713 -0.001713 -0.001713 -0.001713 0 0 0 0.61483 0.61483 0.61483 1 1 1 1.006884 1.006884 1.006884 1.006884
  spline S89 degree 3 poles (90.6552, -5.8065) (90.657, -5.7996) (90.6588, -5.7926) (90.6607, -5.7856) (90.733, -5.5087) (90.8262, -5.1272) (90.8895, -4.6883) (90.9554, -4.2319) (90.9752, -3.8126) (90.9833, -3.46) (90.9871, -3.2972) (90.9887, -3.1396) (90.9899, -2.97) (90.9899, -2.9637) (90.99, -2.9575) (90.99, -2.9512) knots -0.013642 -0.013642 -0.013642 -0.013642 0 0 0 0.396848 0.396848 0.396848 0.809537 0.809537 0.809537 1 1 1 1.007635 1.007635 1.007635 1.007635
  spline S90 degree 3 poles (90.99, -2.9512) (90.99, -2.945) (90.99, -2.9387) (90.99, -2.9324) (90.99, -2.4724) (90.9918, -2.0648) (90.9385, -1.5182) (90.894, -1.0612) (90.7945, -0.5524) (90.7035, -0.1972) knots -0.008156 -0.008156 -0.008156 -0.008156 0 0 0 0.542171 0.542171 0.542171 0.995571 0.995571 0.995571 0.995571
  spline S91 degree 3 poles (90.7035, -0.1972) (90.0207, 2.4927) (88.4137, 4.7645) (86.3566, 6.2808) (84.0823, 7.9571) (81.2395, 8.778) (78.3374, 8.4691) (76.8124, 8.3068) (75.2779, 7.8223) (73.8742, 7.0139) (73.8718, 7.0125) (73.8695, 7.0112) (73.8671, 7.0098) knots 0.000464 0.000464 0.000464 0.000464 0.372519 0.372519 0.372519 0.783863 0.783863 0.783863 1 1 1 1.000666 1.000666 1.000666 1.000666
  spline S92 degree 3 poles (73.8671, 7.0098) (73.8648, 7.0085) (73.8624, 7.0071) (73.8601, 7.0058) (73.3872, 6.7315) (72.5139, 6.4068) (71.5763, 6.2647) (71.5754, 6.2646) (71.5746, 6.2645) (71.5738, 6.2644) knots -0.002014 -0.002014 -0.002014 -0.002014 0 0 0 1 1 1 1.000529 1.000529 1.000529 1.000529
  spline S93 degree 3 poles (71.5738, 6.2644) (71.573, 6.2642) (71.5722, 6.2641) (71.5714, 6.264) (71.3614, 6.232) (71.2742, 6.2187) (70.8167, 6.196) (69.9643, 6.1538) (68.0415, 6.1301) (63.8076, 6.1296) (61.8513, 6.1294) (59.3936, 6.1329) (56.2898, 6.1383) (56.2895, 6.1383) (56.2893, 6.1383) (56.289, 6.1383) knots -0.000626 -0.000626 -0.000626 -0.000626 0 0 0 0.268512 0.268512 0.268512 0.768828 0.768828 0.768828 1 1 1 1.000018 1.000018 1.000018 1.000018
  spline S94 degree 3 poles (56.289, 6.1383) (56.2888, 6.1383) (56.2885, 6.1383) (56.2883, 6.1383) (49.3494, 6.1484) (45.9764, 6.157) (44.3196, 6.178) (43.4713, 6.1887) (43.0795, 6.2058) (42.9969, 6.2117) knots -0.000021 -0.000021 -0.000021 -0.000021 0 0 0 0.57731 0.57731 0.57731 0.872881 0.872881 0.872881 0.872881
  spline S95 degree 3 poles (42.9969, 6.2117) (41.7382, 6.3892) (40.8689, 6.7147) (40.3346, 7.028) (40.3327, 7.0292) (40.3307, 7.0303) (40.3287, 7.0315) knots 0.011769 0.011769 0.011769 0.011769 1 1 1 1.001555 1.001555 1.001555 1.001555
  spline S96 degree 3 poles (40.3287, 7.0315) (40.3267, 7.0327) (40.3247, 7.0338) (40.3227, 7.035) (38.6981, 7.9819) (36.9979, 8.4238) (35.2421, 8.5141) (34.6806, 8.5429) (34.1121, 8.532) (33.5366, 8.4758) knots -0.001959 -0.001959 -0.001959 -0.001959 0 0 0 0.757667 0.757667 0.757667 1 1 1 1
  spline S97 degree 3 poles (33.5366, 8.4758) (30.8677, 8.2168) (28.5164, 7.0321) (26.7116, 5.2837) (25.4993, 4.1093) (24.5193, 2.6566) (23.9141, 0.9718) (23.9134, 0.9701) (23.9128, 0.9684) (23.9122, 0.9667) knots 0.000479 0.000479 0.000479 0.000479 0.598384 0.598384 0.598384 1 1 1 1.000779 1.000779 1.000779 1.000779
  spline S98 degree 3 poles (23.9122, 0.9667) (23.9116, 0.965) (23.911, 0.9633) (23.9104, 0.9616) (23.0138, -1.5501) (23.0115, -4.3472) (23.9141, -6.8271) (24.4359, -8.2609) (25.2452, -9.5852) (26.2718, -10.7258) (26.2719, -10.726) (26.272, -10.7261) (26.2722, -10.7263) knots -0.000763 -0.000763 -0.000763 -0.000763 0 0 0 0.633646 0.633646 0.633646 1 1 1 1.000083 1.000083 1.000083 1.000083
  spline S99 degree 3 poles (26.2722, -10.7263) (26.2723, -10.7264) (26.2725, -10.7266) (26.2726, -10.7267) (26.5124, -10.993) (26.9944, -11.7509) (27.3817, -13.0097) (27.5196, -13.4579) (27.6479, -13.9658) (27.7595, -14.5271) (27.7597, -14.5281) (27.7599, -14.5292) (27.7601, -14.5302) knots -0.000107 -0.000107 -0.000107 -0.000107 0 0 0 0.737392 0.737392 0.737392 1 1 1 1.000384 1.000384 1.000384 1.000384
  line L60 (27.7601, -14.5302) -> (27.7929, -14.694)
  line L61 (27.7929, -14.694) -> (27.8208, -26.7737)
  line L62 (27.8208, -26.7737) -> (27.8515, -40.0619)
  line L63 (27.8515, -40.0619) -> (28.1853, -41.3106)
  line L64 (43.2375, -50.3785) -> (41.2195, -50.3427)
  line L65 (41.3067, -51.183) -> (40.09, -51.1135)
  dimension "d3" = 4.5
  dimension "d4" = 5.3
  constraint coincident S60 L64.end
  constraint coincident S81 L65.end
extrude "Extrude2" add sketch "Sketch2" against normal blind 5 separate body makes body 2 at (49.6117, 0, 50.8973) makes body 3 at (81.3493, 0, 2.502)